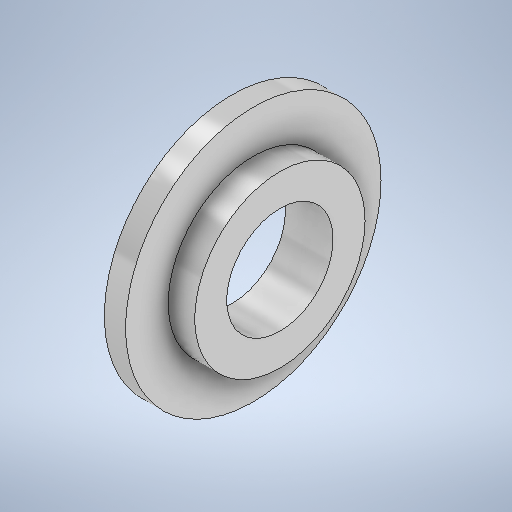
# Autodesk Inventor part: 04
Saved by Autodesk Inventor 2025.1 (Build 291241000, 241)
## iProperties
Created: 2024-09-17
Part Number: 04
Material: Aluminum 6061
Document SubType Name: Modeling
Designer: ffogue
Density: 2.7 g/cm^3
Appearance: Aluminum - Polished
Author: ffogue
Autodesk Inventor part; units mm, degrees
ref_plane "YZ Plane" through (0, 0, 0) normal (1, 0, 0) x (0, 1, 0)
ref_plane "XZ Plane" through (0, 0, 0) normal (0, 1, 0) x (-1, 0, 0)
ref_plane "XY Plane" through (0, 0, 0) normal (0, 0, 1) x (1, 0, 0)
sketch "Sketch1" plane through (0, 0, 0) normal (0, 0, 1) x (1, 0, 0)
  line L0 (0, 0) -> (0, 12)
  line L1 (0, 12) -> (2, 12)
  line L2 (2, 12) -> (2, 8)
  line L3 (2, 8) -> (4.5, 8)
  line L4 (4.5, 8) -> (4.5, 0)
  line L5 (4.5, 0) -> (0, 0)
  dimension "d0" = 2.5
  dimension "d1" = 2
  dimension "d2" = 24
  dimension "d3" = 16
  constraints: 12 end point, 5 perpendicular, 1 vertical
  measures "d0" distance of L2.end L3.end
  measures "d1" distance of L0.end L1.end
  measures "d2" diameter of L1 L5
  measures "d3" diameter of L3 L5
revolve "Revolution1" add sketch "Sketch1" angle 360 about axis through (4.5, 0, 0) along (-1, 0, 0)
sketch "Sketch2" plane through (4.5, 0, 0) normal (1, 0, 0) x (0, 0, -1)
  circle A0 centre (0, 0) radius 8 projected
  point P0 (0, 0)
  constraints: 1 coincident
hole "Hole1" at (4.5, 0, 0) direction (-1, 0, 0) diameter 10 depth 4.5
body "Solid1"
